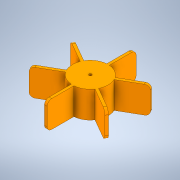
# Autodesk Inventor part: sketch_for_propeller
Saved by Autodesk Inventor 2021 (Build 250183000, 183)
## iProperties
Created: 2023-05-04
Part Number: sketch_for_propeller
Material: Generic
Document SubType Name: Modeling
Designer: assman
Density: 1 g/cm^3
Appearance: Default
Author: assman
Autodesk Inventor part; units mm, degrees
ref_plane "YZ Plane" through (0, 0, 0) normal (1, 0, 0) x (0, 1, 0)
ref_plane "XZ Plane" through (0, 0, 0) normal (0, 1, 0) x (-1, 0, 0)
ref_plane "XY Plane" through (0, 0, 0) normal (0, 0, 1) x (1, 0, 0)
sketch "Sketch1" plane through (0, 0, 0) normal (0, 1, 0) x (-1, 0, 0)
  line L0 (0, 50) -> (0, 20) construction
  line L1 (0, -20) -> (0, -50) construction
  line L2 (-43.3013, 25) -> (-17.3205, 10) construction
  line L3 (18.0217, -8.6728) -> (44.0318, -23.6897) construction
  line L4 (-43.3013, -25) -> (-17.3205, -10) construction
  line L5 (17.3205, 10) -> (43.3013, 25) construction
  line L6 (-1.5, -19.9437) -> (-1.5, -49.9775)
  line L7 (1.5, -19.9437) -> (1.5, -49.9775)
  line L8 (-44.0318, -23.6897) -> (-18.0217, -8.6728)
  line L9 (-42.5318, -26.2878) -> (-16.5217, -11.2709)
  line L10 (-44.0318, 23.6897) -> (-18.0217, 8.6728)
  line L11 (-42.5318, 26.2878) -> (-16.5217, 11.2709)
  line L12 (-1.5, 49.9775) -> (-1.5, 19.9437)
  line L13 (1.5, 49.9775) -> (1.5, 19.9437)
  line L14 (16.5217, 11.2709) -> (42.5318, 26.2878)
  line L15 (18.0217, 8.6728) -> (44.0318, 23.6897)
  line L16 (17.3205, -10) -> (43.3013, -25)
  line L17 (18.6245, -7.2888) -> (44.7233, -22.3569)
  arc A0 (-1.5, -49.9775) -> (1.5, -49.9775) centre (0, 0) ccw
  arc A1 (-44.0318, -23.6897) -> (-42.5318, -26.2878) centre (0, 0) ccw
  arc A2 (-42.5318, 26.2878) -> (-44.0318, 23.6897) centre (0, 0) ccw
  arc A3 (1.5, 49.9775) -> (-1.5, 49.9775) centre (0, 0) ccw
  arc A4 (43.3013, -25) -> (44.7233, -22.3569) centre (0, 0) ccw
  arc A5 (44.0318, 23.6897) -> (42.5318, 26.2878) centre (0, 0) ccw
  arc A6 (16.5217, 11.2709) -> (1.5, 19.9437) centre (0, 0) ccw
  arc A7 (18.6245, -7.2888) -> (18.0217, 8.6728) centre (0, 0) ccw
  arc A8 (1.5, -19.9437) -> (17.3205, -10) centre (0, 0) ccw
  arc A9 (-16.5217, -11.2709) -> (-1.5, -19.9437) centre (0, 0) ccw
  arc A10 (-1.5, 19.9437) -> (-16.5217, 11.2709) centre (0, 0) ccw
  arc A11 (-18.0217, 8.6728) -> (-18.0217, -8.6728) centre (0, 0) ccw
  dimension "d8" = 1.5
  dimension "d9" = 1.5
  dimension "d10" = 1.5
  dimension "d11" = 1.5
  dimension "d12" = 1.5
  dimension "d13" = 1.5
  dimension "d14" = 1.5
  dimension "d15" = 1.5
  dimension "d16" = 1.5
  dimension "d17" = 1.5
  dimension "d18" = 1.5
  dimension "d19" = 1.5
  constraints: 36 end point, 30 point on circle, 12 centre point, 12 parallel, 2 coincident, 2 vertical
  measures "d8" distance between parallel lines of L1 L6
  measures "d9" distance between parallel lines of L1 L7
  measures "d10" distance between parallel lines of L4 L8
  measures "d11" distance between parallel lines of L4 L9
  measures "d12" distance between parallel lines of L2 L10
  measures "d13" distance between parallel lines of L2 L11
  measures "d14" distance between parallel lines of L0 L12
  measures "d15" distance between parallel lines of L0 L13
  measures "d16" distance between parallel lines of L5 L14
  measures "d17" distance between parallel lines of L5 L15
  measures "d18" distance between parallel lines of L3 L16
  measures "d19" distance between parallel lines of L3 L17
extrude "Extrusion1" add sketch "Sketch1" along normal blind 30
fillet "Fillet1" radius 5 12 edges at (-43.3013, 30, 25) (-43.3013, 0, 25) (-44.0321, 30, -23.6891) (-44.0321, 0, -23.6891) (0, 30, 50) (0, 0, 50) (43.3013, 0, 25) (43.3013, 30, 25) (43.3013, 30, -25) (43.3013, 0, -25) (0, 30, -50) (0, 0, -50)
sketch "Sketch2" plane through (0, 30, 0) normal (0, 1, 0) x (1, 0, 0)
  arc A0 (1.5, 44.975) -> (-1.5, 44.975) centre (0, 0) ccw construction
  line L0 (-1.5, 44.975) -> (-1.5, 19.9437) construction
  arc A1 (-1.5, 19.9437) -> (-17.3205, 10) centre (0, 0) ccw construction
  line L1 (-17.3205, 10) -> (-38.9711, 22.5) construction
  arc A2 (-38.9711, 22.5) -> (-40.3844, 19.8519) centre (0, 0) ccw construction
  line L2 (-40.3844, 19.8519) -> (-18.6245, 7.2888) construction
  arc A3 (-18.6245, 7.2888) -> (-18.0217, -8.6728) centre (0, 0) ccw construction
  line L3 (-18.0217, -8.6728) -> (-39.6995, -21.1885) construction
  arc A4 (-39.6995, -21.1885) -> (-38.1995, -23.7865) centre (0, 0) ccw construction
  line L4 (-38.1995, -23.7865) -> (-16.5217, -11.2709) construction
  arc A5 (-16.5217, -11.2709) -> (-1.5, -19.9437) centre (0, 0) ccw construction
  line L5 (-1.5, -19.9437) -> (-1.5, -44.975) construction
  arc A6 (-1.5, -44.975) -> (1.5, -44.975) centre (0, 0) ccw construction
  line L6 (1.5, -44.975) -> (1.5, -19.9437) construction
  arc A7 (1.5, -19.9437) -> (16.5217, -11.2709) centre (0, 0) ccw construction
  line L7 (16.5217, -11.2709) -> (38.1995, -23.7865) construction
  arc A8 (38.1995, -23.7865) -> (39.6995, -21.1885) centre (0, 0) ccw construction
  line L8 (39.6995, -21.1885) -> (18.0217, -8.6728) construction
  arc A9 (18.0217, -8.6728) -> (18.0217, 8.6728) centre (0, 0) ccw construction
  line L9 (18.0217, 8.6728) -> (39.6995, 21.1885) construction
  arc A10 (39.6995, 21.1885) -> (38.1995, 23.7865) centre (0, 0) ccw construction
  line L10 (38.1995, 23.7865) -> (16.5217, 11.2709) construction
  arc A11 (16.5217, 11.2709) -> (1.5, 19.9437) centre (0, 0) ccw construction
  line L11 (1.5, 19.9437) -> (1.5, 44.975) construction
  circle A12 centre (0, 0) radius 1.5
  dimension "d23" = 3
  constraints: 1 centre point, 1 coincident
  measures "d23" diameter of A12
extrude "Extrusion2" cut sketch "Sketch2" against normal blind 5
equation "\"d8\" = 0.5 * blade_width"
equation "\"d9\" = 0.5 * blade_width"
equation "\"d10\" = 0.5 * blade_width"
equation "\"d11\" = 0.5 * blade_width"
equation "\"d12\" = 0.5 * blade_width"
equation "\"d13\" = 0.5 * blade_width"
equation "\"d14\" = 0.5 * blade_width"
equation "\"d15\" = 0.5 * blade_width"
equation "\"d16\" = 0.5 * blade_width"
equation "\"d17\" = 0.5 * blade_width"
equation "\"d18\" = 0.5 * blade_width"
equation "\"d19\" = 0.5 * blade_width"
equation "\"d20\" = blade_height"
equation "\"blade_width\" = 3"
equation "\"blade_height\" = 30"
body "Solid1"
